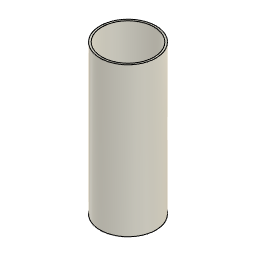
Main Body v4 (Autodesk Fusion 360 design; units mm, degrees)
Autodesk Fusion 360 part; units mm, degrees
sketch "Sketch1" plane through (0, 0, 0) normal (1, 0, 0) x (0, 1, 0)
  line L0 (30, 0) -> (30, 160)
  line L1 (30, 160) -> (28, 160)
  line L2 (28, 160) -> (28, 0)
  line L3 (28, 0) -> (30, 0)
  dimension "d1" = 30
  dimension "d2" = 160
  dimension "d3" = 2
  constraint horizontal L1
  measures "d1" distance of origin L0.start
  measures "d2" distance of L0.start L0.end
  measures "d3" distance of L0.end L1.end
revolve "Revolve1" add sketch "Sketch1" angle 360 about axis through (0, 0, 1.75) along (0, 0, 1)
